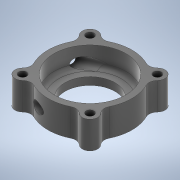
# Autodesk Inventor part: Case
Saved by Autodesk Inventor 2020.2 (Build 242310000, 310)
## iProperties
Created: 2020-09-02
Part Number: Case
Material: Generic
Document SubType Name: Modeling
Designer: JK
Density: 1 g/cm^3
Appearance: Smooth - Black
Author: JK
Autodesk Inventor part; units mm, degrees
ref_plane "YZ Plane" through (0, 0, 0) normal (1, 0, 0) x (0, 1, 0)
ref_plane "XZ Plane" through (0, 0, 0) normal (0, 1, 0) x (-1, 0, 0)
sketch "Sketch1" plane through (0, 0, 0) normal (0, 1, 0) x (-1, 0, 0)
  line L0 (-21, 21) -> (21, 21)
  line L1 (21, 21) -> (21, -21)
  line L2 (21, -21) -> (-21, -21)
  line L3 (-21, -21) -> (-21, 21)
  line L4 (-21, 21) -> (21, -21) construction
  line L5 (21, 21) -> (-21, -21) construction
  circle A0 centre (15.5, 15.5) radius 1.8
  circle A1 centre (15.5, -15.5) radius 1.8
  circle A2 centre (-15.5, -15.5) radius 1.8
  circle A3 centre (-15.5, 15.5) radius 1.8
  circle A4 centre (0, 0) radius 11.5
  dimension "d0" = 3.6
  dimension "d1" = 42
  dimension "d2" = 42
  dimension "d3" = 31
  dimension "d4" = 23
  constraints: 12 end point, 5 centre point, 4 point on line, 3 equal radius, 2 midpoint, 2 parallel, 2 vertical alignment, 1 coincident, 1 horizontal, 1 horizontal alignment, 1 perpendicular
  measures "d0" diameter of A0
  measures "d1" distance of L0.end L1.end
  measures "d2" distance of L1.end L2.end
  measures "d3" distance of A1.centre A0.centre
  measures "d4" diameter of A4
extrude "Extrusion1" add sketch "Sketch1" along normal blind 2.5
sketch "Sketch2" plane through (0, 2.5, 0) normal (0, 1, 0) x (1, 0, 0)
  circle A0 centre (0, 0) radius 19.3
  circle A1 centre (0, 0) radius 16.5
  dimension "d7" = 2.8
  dimension "d8" = 33
  constraints: 2 centre point, 2 coincident
  measures "d7" radial gap between concentric circles of A0 A1
  measures "d8" diameter of A1
extrude "Extrusion2" add sketch "Sketch2" along normal blind 9.1
sketch "Sketch3" plane through (0, 2.5, 0) normal (0, 1, 0) x (1, 0, 0)
  circle A0 centre (-15.5, -15.5) radius 1.8 projected
  circle A1 centre (-15.5, -15.5) radius 3.5
  circle A2 centre (-15.5, -15.5) radius 1.8
  circle A3 centre (0, 0) radius 19.3 projected
  line L0 (-10.946, -15.8958) -> (-13.0251, -17.9749)
  line L1 (-17.9749, -13.0251) -> (-15.8958, -10.946)
  dimension "d11" = 7
  constraints: 4 end point, 4 point on circle, 2 centre point, 2 coincident, 2 parallel, 2 tangent
  measures "d11" diameter of A1
extrude "Extrusion3" add sketch "Sketch3" along normal up to surface (9.1 mm away) contours A1 A3 | L1 A3 A1 | A1 A3 L0 picked at (-14.8438, -12.9535)
pattern_circular "Circular Pattern1" count 4 over 360 about axis through (0, 2.5, 0) along (0, 1, 0) of "Extrusion3"
sketch "Sketch4" plane through (0, 2.5, 0) normal (0, 1, 0) x (1, 0, 0)
  line L0 (-13.0251, 17.9749) -> (-10.946, 15.8958) projected
  arc A0 (10.946, 15.8958) -> (-10.946, 15.8958) centre (0, 0) ccw projected
  line L1 (10.946, 15.8958) -> (13.0251, 17.9749) projected
  arc A1 (17.9749, 13.0251) -> (13.0251, 17.9749) centre (15.5, 15.5) ccw projected
  line L2 (17.9749, 13.0251) -> (15.8958, 10.946) projected
  arc A2 (15.8958, -10.946) -> (15.8958, 10.946) centre (0, 0) ccw projected
  line L3 (15.8958, -10.946) -> (17.9749, -13.0251) projected
  arc A3 (13.0251, -17.9749) -> (17.9749, -13.0251) centre (15.5, -15.5) ccw projected
  line L4 (13.0251, -17.9749) -> (10.946, -15.8958) projected
  arc A4 (-10.946, -15.8958) -> (10.946, -15.8958) centre (0, 0) ccw projected
  line L5 (-10.946, -15.8958) -> (-13.0251, -17.9749) projected
  arc A5 (-17.9749, -13.0251) -> (-13.0251, -17.9749) centre (-15.5, -15.5) ccw projected
  line L6 (-17.9749, -13.0251) -> (-15.8958, -10.946) projected
  arc A6 (-15.8958, 10.946) -> (-15.8958, -10.946) centre (0, 0) ccw projected
  line L7 (-15.8958, 10.946) -> (-17.9749, 13.0251) projected
  arc A7 (-13.0251, 17.9749) -> (-17.9749, 13.0251) centre (-15.5, 15.5) ccw projected
  line L8 (-21, -21) -> (21, -21) projected
  line L9 (21, -21) -> (21, 21) projected
  line L10 (21, 21) -> (-21, 21) projected
  line L11 (-21, 21) -> (-21, -21) projected
extrude "Extrusion4" cut sketch "Sketch4" against normal through all
fillet "Fillet1" radius 2 1 edges at (-16.5, 2.5, 0)
ref_plane "Work Plane1" through (0, 0, 0) normal (0.9063078, 0, -0.4226183) x (0, 1, 0)
sketch "Sketch7" plane through (0, 0, 0) normal (0.9063078, 0, -0.4226183) x (0, 1, 0)
  circle A0 centre (4.8, 14.2) radius 2.3
  circle A1 centre (4.8, -14.2) radius 2.3
  line L0 (2.5, 14.5) -> (2.5, -14.5) projected
  point P0 (0, 0)
  dimension "d24" = 4.6
  dimension "d34" = 14.2
  dimension "d35" = 14.2
  constraints: 2 centre point, 1 equal radius, 1 tangent, 1 vertical alignment
  measures "d24" diameter of A0
  measures "d34" vertical distance of point (0, 0) A0.centre
  measures "d35" vertical distance of A1.centre point (0, 0)
extrude "Extrusion5" cut sketch "Sketch7" against normal blind 25.5
fillet "Fillet3" radius 4 14 edges at (-10.946, 5.8, -15.8958) (10.946, 5.8, -15.8958) (15.8958, 7.05, -10.946) (15.8958, 1.25, -10.946) (15.8958, 7.05, 10.946) (15.8958, 1.25, 10.946) (10.946, 7.05, 15.8958) (10.946, 1.25, 15.8958) (-10.946, 7.05, 15.8958) (-10.946, 1.25, 15.8958) (-15.8958, 7.05, 10.946) (-15.8958, 1.25, 10.946) (-15.8958, 7.05, -10.946) (-15.8958, 1.25, -10.946)
sketch "Sketch8" plane through (0, 0, 0) normal (0, -1, 0) x (1, 0, 0)
  arc A0 (13.0718, -18.0207) -> (18.0207, -13.0718) centre (15.5, -15.5) ccw projected
  arc A1 (17.3132, -8.529) -> (17.3132, 8.529) centre (0, 0) ccw projected
  arc A2 (18.0207, 13.0718) -> (13.0718, 18.0207) centre (15.5, 15.5) ccw projected
  arc A3 (8.529, 17.3132) -> (-8.529, 17.3132) centre (0, 0) ccw projected
  arc A4 (-13.0718, 18.0207) -> (-18.0207, 13.0718) centre (-15.5, 15.5) ccw projected
  arc A5 (-17.3132, 8.529) -> (-17.3132, -8.529) centre (0, 0) ccw projected
  arc A6 (-18.0207, -13.0718) -> (-13.0718, -18.0207) centre (-15.5, -15.5) ccw projected
  arc A7 (-8.529, -17.3132) -> (8.529, -17.3132) centre (0, 0) ccw projected
  circle A8 centre (0, 0) radius 11.5 projected
  circle A9 centre (15.5, 15.5) radius 1.8 projected
  circle A10 centre (15.5, -15.5) radius 1.8 projected
  circle A11 centre (-15.5, -15.5) radius 1.8 projected
  circle A12 centre (-15.5, 15.5) radius 1.8 projected
  arc A13 (-13.0718, 18.0207) -> (-8.529, 17.3132) centre (-10.2967, 20.9014) ccw projected
  arc A14 (-17.3132, 8.529) -> (-18.0207, 13.0718) centre (-20.9014, 10.2967) ccw projected
  arc A15 (-18.0207, -13.0718) -> (-17.3132, -8.529) centre (-20.9014, -10.2967) ccw projected
  arc A16 (-8.529, -17.3132) -> (-13.0718, -18.0207) centre (-10.2967, -20.9014) ccw projected
  arc A17 (13.0718, -18.0207) -> (8.529, -17.3132) centre (10.2967, -20.9014) ccw projected
  arc A18 (17.3132, -8.529) -> (18.0207, -13.0718) centre (20.9014, -10.2967) ccw projected
  arc A19 (18.0207, 13.0718) -> (17.3132, 8.529) centre (20.9014, 10.2967) ccw projected
  arc A20 (8.529, 17.3132) -> (13.0718, 18.0207) centre (10.2967, 20.9014) ccw projected
extrude "Extrusion6" add sketch "Sketch8" along normal blind 1
body "Solid1"
